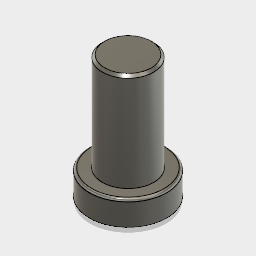
stamp (Autodesk Fusion 360 design; units mm, degrees)
Autodesk Fusion 360 part; units mm, degrees
cylinder "CylinderPrimitive1" add diameter 25 height 50 placed x (1, 0, 0) y (0, 0, -1) z (0, 1, 0) at (0, 0, 0)
sketch "Sketch3" plane through (0, 0, 0) normal (0, 1, 0) x (1, 0, 0)
sketch "Sketch4" plane through (0, 0, 0) normal (0, 1, 0) x (1, 0, 0)
  circle A0 centre (0, 0) radius 15.8114
extrude "Extrude1" add sketch "Sketch4" along normal blind 10
sketch "Sketch5" plane through (0, 0, 0) normal (0, -1, 0) x (1, 0, 0)
  circle A0 centre (0, 0) radius 15.8114
  circle A1 centre (0, 0) radius 12.8114
  ellipse E0 centre (-7.9413, 2.9586) end of major axis (-6.5576, -0.0829) minor radius 2.2602
  line L0 (-9.325, 6) -> (-6.5576, -0.0829)
  line L1 (-9.9986, 2.0226) -> (-5.884, 3.8946)
  ellipse E1 centre (-2.904, 6.9397) end of major axis (-2.0694, 3.7042) minor radius 2.2602
  ellipse E2 centre (3.463, 6.6881) end of major axis (3.1406, 3.3623) minor radius 2.2602
  ellipse E3 centre (8.3894, 2.5523) end of major axis (7.4944, -0.667) minor radius 2.2602
  line L2 (-2.8087, -10.6818) -> (0, -10)
  line L3 (0, -10) -> (3.3296, -10.5961)
  line L4 (-3.3849, 0) -> (-5, -2.1517)
  line L5 (-5, -2.1517) -> (-6.6153, -3.6803)
  line L6 (3.2101, 0) -> (5.2463, -2.1517)
  line L7 (5.2463, -2.1517) -> (6.7092, -3.3813)
  arc A2 (-6.6153, -3.6803) -> (-2.8087, -10.6818) centre (-3.7813, -6.675) ccw
  arc A3 (3.2101, 0) -> (-3.3849, 0) centre (-0.0874, -2.4752) ccw
  arc A4 (-0.0664, -6.5982) -> (0.3406, -6.576) centre (-0.0874, -2.4752) ccw
  arc A5 (3.3296, -10.5961) -> (6.7092, -3.3813) centre (4.0562, -6.5376) ccw
  dimension "d5" = 3
extrude "Extrude2" cut sketch "Sketch5" against normal blind 2 contours A1
sketch "Sketch6" plane through (0, 0, 0) normal (0, 0, 1) x (1, 0, 0)
fillet "Fillet1" radius 1 1 edges at (-14.7414, 10, 5.7176)
extrude "Extrude3" add 1 faces at (-0.5966, 0, -4.0506) along direction (0, -1, 0) blind 2
extrude "Extrude4" add 1 faces at (9.0826, 0, 2.2492) along direction (0, -1, 0) blind 2
extrude "Extrude5" add 1 faces at (4.1983, 0, 6.51) along direction (0, -1, 0) blind 2
extrude "Extrude6" add 1 faces at (-2.152, 0, 7.0238) along direction (0, -1, 0) blind 2
extrude "Extrude7" add 1 faces at (-7.4205, 0, 3.607) along direction (0, -1, 0) blind 2
extrude "Extrude8" add 1 faces at (-9.1319, 2, -2.6355) along direction (0, -1, 0) blind 2
chamfer "Chamfer1" distance 1 angle 45 1 edges at (-11.6541, 50, 4.5202)
move_face "OffsetFaces1" offset -2 1 faces at (12.4379, 36, 1.2446)
